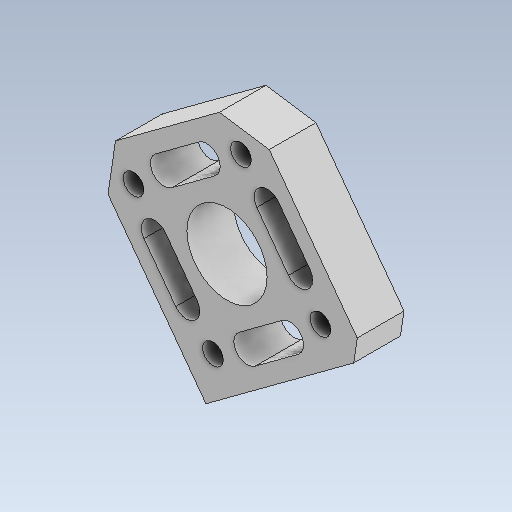
# Autodesk Inventor part: slide_holder_3
Saved by Autodesk Inventor 2020 (Build 240168000, 168)
## iProperties
Created: 2020-05-14
Part Number: slide_holder_3
Material: Generic
Document SubType Name: Modeling
Designer: psrobotics
Density: 1 g/cm^3
Appearance: Default
Author: psrobotics
Autodesk Inventor part; units mm, degrees
ref_plane "YZ Plane" through (0, 0, 0) normal (1, 0, 0) x (0, 1, 0)
ref_plane "XZ Plane" through (0, 0, 0) normal (0, 1, 0) x (-1, 0, 0)
ref_plane "XY Plane" through (0, 0, 0) normal (0, 0, 1) x (1, 0, 0)
sketch "Sketch1" plane through (0, 0, 0) normal (0, 0, 1) x (1, 0, 0)
  arc A0 (-0.864, -1.0803) -> (2.3529, 1.2971) centre (0.7444, 0.1084) ccw projected
  line L0 (-0.864, -1.0803) -> (-5.6188, 5.3534) projected
  arc A1 (-2.4019, 7.7308) -> (-5.6188, 5.3534) centre (-4.0104, 6.5421) ccw projected
  line L1 (-2.4019, 7.7308) -> (2.3529, 1.2971) projected
  line L2 (11.4273, 9.6732) -> (1.4127, 12.4362) projected
  arc A2 (1.0876, 16.1712) -> (1.4127, 12.4362) centre (1.9446, 14.3641) ccw projected
  line L3 (1.0876, 16.1712) -> (6.3388, 18.6615) projected
  arc A3 (8.6773, 18.1979) -> (6.3388, 18.6615) centre (7.1957, 16.8544) ccw projected
  line L4 (8.6773, 18.1979) -> (13.4408, 12.9447) projected
  arc A4 (11.4273, 9.6732) -> (13.4408, 12.9447) centre (11.9592, 11.6012) ccw projected
  line L5 (-16.3374, -3.2308) -> (-6.1076, -6.0531) projected
  arc A5 (-5.7826, -9.7881) -> (-6.1076, -6.0531) centre (-6.6396, -7.981) ccw projected
  line L6 (-5.7826, -9.7881) -> (-11.1465, -12.3319) projected
  arc A6 (-13.4851, -11.8683) -> (-11.1465, -12.3319) centre (-12.0035, -10.5248) ccw projected
  line L7 (-13.4851, -11.8683) -> (-18.3509, -6.5022) projected
  arc A7 (-16.3374, -3.2308) -> (-18.3509, -6.5022) centre (-16.8694, -5.1588) ccw projected
  line L8 (16.896, -0.2335) -> (11.8169, -2.6422) projected
  arc A8 (9.0382, -1.3892) -> (11.8169, -2.6422) centre (10.9599, -0.8351) ccw projected
  line L9 (9.0382, -1.3892) -> (7.8446, 2.75) projected
  arc A9 (10.2983, 5.2321) -> (7.8446, 2.75) centre (9.7663, 3.3041) ccw projected
  line L10 (10.2983, 5.2321) -> (16.5709, 3.5016) projected
  arc A10 (16.896, -0.2335) -> (16.5709, 3.5016) centre (16.039, 1.5736) ccw projected
  line L11 (-15.8844, 1.1079) -> (-21.1286, 2.5547) projected
  arc A11 (-21.4537, 6.2897) -> (-21.1286, 2.5547) centre (-20.5967, 4.4826) ccw projected
  line L12 (-21.4537, 6.2897) -> (-17.2074, 8.3035) projected
  arc A12 (-14.4287, 7.0505) -> (-17.2074, 8.3035) centre (-16.3504, 6.4964) ccw projected
  line L13 (-14.4287, 7.0505) -> (-13.4308, 3.59) projected
  arc A13 (-15.8844, 1.1079) -> (-13.4308, 3.59) centre (-15.3525, 3.0358) ccw projected
  circle A14 centre (-7.0542, 0.7543) radius 1.5 projected
  circle A15 centre (4.3105, -4.7168) radius 1.5 projected
  circle A16 centre (3.7883, 5.8962) radius 1.5 projected
  circle A17 centre (-7.5764, 11.3673) radius 1.5 projected
  line L14 (-32.8464, -33.5183) -> (-37.042, -32.8888) projected
  line L15 (-32.8464, -33.5183) -> (-11.1328, -17.4709) projected
  line L16 (-11.1328, -17.4709) -> (24.3962, -0.6219) projected
  line L17 (24.3962, -0.6219) -> (46.914, 16.0199) projected
  line L18 (47.5436, 20.2156) -> (46.914, 16.0199) projected
  line L19 (47.5436, 20.2156) -> (33.2792, 39.5165) projected
  line L20 (29.0835, 40.1461) -> (33.2792, 39.5165) projected
  line L21 (29.0835, 40.1461) -> (6.5657, 23.5043) projected
  line L22 (6.5657, 23.5043) -> (-28.9633, 6.6553) projected
  line L23 (-28.9633, 6.6553) -> (-50.6769, -9.3921) projected
  line L24 (-51.3064, -13.5878) -> (-50.6769, -9.3921) projected
  line L25 (-51.3064, -13.5878) -> (-37.042, -32.8888) projected
  circle A18 centre (-30.0126, -0.3375) radius 2.05 projected
  circle A19 centre (-18.1256, -16.4216) radius 2.05 projected
  circle A20 centre (13.9606, 22.7522) radius 2.05 projected
  circle A21 centre (41.9318, 18.5551) radius 2.05 projected
  circle A22 centre (25.8476, 6.6681) radius 2.05 projected
  circle A23 centre (30.0448, 34.6392) radius 2.05 projected
  circle A24 centre (-34.2097, -28.3086) radius 2.05 projected
  circle A25 centre (-46.0967, -12.2245) radius 2.05 projected
  circle A26 centre (-32.1111, -14.323) radius 8 projected
  circle A27 centre (27.9462, 20.6536) radius 8 projected
  circle A28 centre (27.9462, 20.6536) radius 6
  line L26 (31.4962, 41.9292) -> (49.3266, 17.803)
  line L27 (49.3266, 17.803) -> (24.3962, -0.6219)
  line L28 (24.3962, -0.6219) -> (6.5657, 23.5043)
  line L29 (6.5657, 23.5043) -> (31.4962, 41.9292)
  line L30 (31.4962, 41.9292) -> (24.3962, -0.6219) construction
  line L31 (49.3266, 17.803) -> (6.5657, 23.5043) construction
  point P0 (0, 0)
  dimension "d0" = 12
  dimension "d1" = 30
  dimension "d2" = 31
  constraints: 12 end point, 2 midpoint, 2 parallel, 1 centre point, 1 coincident, 1 collinear, 1 perpendicular
  measures "d0" diameter of A28
  measures "d1" distance of L26.start L26.end
  measures "d2" distance of L26.end L27.end
ref_plane "Work Plane1" through (-59.9905, -97.7914, 7) normal (0, 0, -1) x (0.1483917, 0.9889287, 0)
extrude "Extrusion1" add sketch "Sketch1" along normal up to surface (7 mm away) contours L28 L21 L20 L19 L18 L17 | A27
sketch "Sketch2" plane through (24.3962, -0.6219, 7) normal (0, 0, 1) x (0.8042069, 0.5943494, 0)
  circle A0 centre (25.5, 5) radius 2.05 projected
  circle A1 centre (25.5, 25) radius 2.05 projected
  circle A2 centre (5.5, 25) radius 2.05 projected
  circle A3 centre (5.5, 5) radius 2.05 projected
  circle A4 centre (15.5, 15) radius 6 projected
  line L0 (28, 30) -> (0, 30) projected
  line L1 (0, 30) -> (0, 0) projected
  line L2 (0, 0) -> (28, 0) projected
  line L3 (28, 0) -> (31, 3) projected
  line L4 (31, 3) -> (31, 27) projected
  line L5 (31, 27) -> (28, 30) projected
  line L6 (5.5, 25) -> (25.5, 25)
  line L7 (25.5, 25) -> (25.5, 5)
  line L8 (25.5, 5) -> (5.5, 5)
  line L9 (5.5, 5) -> (5.5, 25)
  line L10 (15.5, 25) -> (15.5, 25.5)
  line L11 (11.5, 25.5) -> (19.5, 25.5) construction
  line L12 (11.5, 23.5) -> (19.5, 23.5)
  line L13 (19.5, 27.5) -> (11.5, 27.5)
  arc A5 (11.5, 27.5) -> (11.5, 23.5) centre (11.5, 25.5) ccw
  arc A6 (19.5, 23.5) -> (19.5, 27.5) centre (19.5, 25.5) ccw
  point P0 (-19.25, 15)
  dimension "d5" = 0.5
  dimension "d6" = 4
  dimension "d7" = 4
  constraints: 18 end point, 4 parallel, 4 point on circle, 4 tangent, 2 centre point, 2 midpoint, 1 horizontal, 1 perpendicular, 1 vertical
  measures "d5" distance of L10.start L10.end
  measures "d6" distance of L10.end L11.end
  measures "d7" diameter of A6
extrude "Extrusion2" cut sketch "Sketch2" against normal blind 10 contours A6 L12 A5 L6 | L6 A5 L13 A6
pattern_circular "Circular Pattern1" count 4 over 360 about axis through (27.9462, 20.6536, 0) along (0, 0, 1) of "Extrusion2"
chamfer "Chamfer1" distance 3 angle 45 1 edges at (6.5657, 23.5043, 3.5)
thicken "Thicken1" operation add thickness 0.5 both sides no extend neighbours yes toward (-0.9870503, 0.1604113, 0) faces at (27.8711, 6.3392, 4.6667)
thicken "Thicken2" operation add thickness 0.5 both sides no extend neighbours yes toward (-0.9967573, -0.0804666, 0) faces at (16.004, 22.9172, 2.3333)
thicken "Thicken3" operation add thickness 0.5 both sides no extend neighbours yes toward (-0.9967573, -0.0804666, 0) faces at (43.9751, 18.72, 2.3333)
thicken "Thicken4" operation add thickness 0.5 both sides no extend neighbours yes toward (-0.9967573, -0.0804666, 0) faces at (32.0881, 34.8042, 2.3333)
thicken "Thicken5" operation add thickness 0.5 both sides no extend neighbours yes toward (0.8042069, 0.5943494, 0) faces at (19.0471, 6.616, 4.6667)
thicken "Thicken6" operation add thickness 0.5 both sides no extend neighbours yes toward (-0.8042069, -0.5943494, 0) faces at (42.7888, 26.6492, 2.3333)
thicken "Thicken7" operation add thickness 2 both sides no extend neighbours yes toward (-0.1483917, -0.9889287, 0) faces at (31.4145, 39.7964, 2.3333)
thicken "Thicken8" operation add thickness 2 both sides no extend neighbours yes toward (0.9889287, -0.1483917, 0) faces at (8.6286, 22.9565, 2.3333)
body "Solid1"
